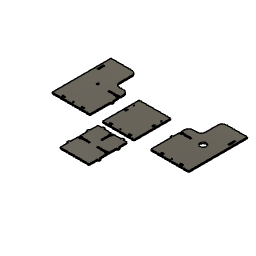
NEW housing (Autodesk Fusion 360 design; units mm, degrees)
Autodesk Fusion 360 part; units mm, degrees
note: some values were not read from the file. Set by a fixed rule: which sketch regions a step uses.
sketch "Sketch1" plane through (0, 0, 0) normal (0, 0, 1) x (1, 0, 0)
  line L0 (-200, 150) -> (-200, 236)
  line L1 (-196, 240) -> (-170, 240)
  line L2 (-160, 230) -> (-160, 225)
  line L3 (-150, 215) -> (-149.9799, 215)
  line L4 (-140, 150) -> (-200, 150)
  arc A0 (-160, 230) -> (-170, 240) centre (-170, 230) ccw
  arc A1 (-160, 225) -> (-150, 215) centre (-150, 225) ccw
  arc A2 (-140, 205) -> (-149.9799, 215) centre (-150, 205) ccw
  arc A3 (-196, 240) -> (-200, 236) centre (-196, 236) ccw
  circle A4 centre (-170, 192.9999) radius 2.5
  line L5 (-140, 205) -> (-140, 204.0941)
  line L6 (-140, 199.6441) -> (-140, 189.8941)
  line L7 (-140, 185.8941) -> (-140, 150)
  line L8 (-155, 153) -> (-155, 154.55)
  line L9 (-155, 154.55) -> (-149, 154.55)
  line L10 (-149, 154.55) -> (-149, 151.45)
  line L11 (-149, 151.45) -> (-155, 151.45)
  line L12 (-155, 151.45) -> (-155, 153)
  line L13 (-185, 153) -> (-185, 154.55)
  line L14 (-185, 154.55) -> (-191, 154.55)
  line L15 (-191, 154.55) -> (-191, 151.45)
  line L16 (-191, 151.45) -> (-185, 151.45)
  line L17 (-185, 151.45) -> (-185, 153)
  circle A5 centre (-170, 153) radius 1.5
  line L18 (-140, 202.9941) -> (-140, 204.0941)
  line L19 (-140, 189.8941) -> (-137.2, 189.8941)
  line L20 (-137.2, 189.8941) -> (-137.2, 185.8941)
  line L21 (-137.2, 185.8941) -> (-140, 185.8941)
  line L22 (-50, 150) -> (10, 150)
  line L23 (-35, 154.55) -> (-41, 154.55)
  line L24 (-52.8, 189.8941) -> (-52.8, 185.8941)
  line L25 (1, 151.45) -> (-5, 151.45)
  line L26 (1, 154.55) -> (1, 151.45)
  arc A6 (-40.0001, 215) -> (-50, 205) centre (-40, 205) ccw
  circle A7 centre (-20, 153) radius 1.5
  line L27 (-5, 154.55) -> (1, 154.55)
  line L28 (-52.8, 185.8941) -> (-50, 185.8941)
  line L29 (-50, 202.9941) -> (-50, 204.0941)
  line L30 (-39.9999, 215) -> (-40.0001, 215)
  line L31 (-41, 154.55) -> (-41, 151.45)
  arc A8 (10, 236) -> (6, 240) centre (6, 236) ccw
  line L32 (-50, 189.8941) -> (-52.8, 189.8941)
  line L33 (-41, 151.45) -> (-35, 151.45)
  line L34 (-50, 205) -> (-50, 204.0941)
  arc A9 (-39.9999, 215) -> (-30, 225) centre (-40, 225) ccw
  arc A10 (-20, 240) -> (-30, 230) centre (-20, 230) ccw
  line L35 (10, 150) -> (10, 236)
  line L36 (-50, 199.6441) -> (-50, 189.8941)
  line L37 (6, 240) -> (-20, 240)
  line L38 (-30, 230) -> (-30, 225)
  line L39 (-35, 153) -> (-35, 154.55)
  line L40 (-5, 153) -> (-5, 154.55)
  line L41 (-35, 151.45) -> (-35, 153)
  line L42 (-50, 185.8941) -> (-50, 150)
  line L43 (-5, 151.45) -> (-5, 153)
  line L44 (-77, 154.55) -> (-71, 154.55)
  line L45 (-77, 153) -> (-77, 154.55)
  line L46 (-77, 151.45) -> (-77, 153)
  line L47 (-71, 151.45) -> (-77, 151.45)
  line L48 (-71, 154.55) -> (-71, 151.45)
  circle A11 centre (-92, 153) radius 1.5
  line L49 (-107, 154.55) -> (-113, 154.55)
  line L50 (-107, 151.45) -> (-107, 153)
  line L51 (-107, 153) -> (-107, 154.55)
  line L52 (-113, 151.45) -> (-107, 151.45)
  line L53 (-113, 154.55) -> (-113, 151.45)
  circle A12 centre (-58.5, 201.1441) radius 1.55
  line L54 (-125, -50) -> (-55, -50)
  line L55 (-110.1464, 10) -> (-110.1464, 12.8)
  line L56 (-110.1464, 12.8) -> (-106, 12.8)
  line L57 (-106, 12.8) -> (-106, 10)
  line L58 (-73.9655, 10) -> (-73.9655, 12.8)
  line L59 (-73.9655, 12.8) -> (-69.9655, 12.8)
  line L60 (-69.9655, 12.8) -> (-69.9655, 10)
  line L61 (-91.55, 10) -> (-106, 10)
  line L62 (-110.1464, 10) -> (-125, 10)
  line L63 (-55, 10) -> (-69.9655, 10)
  line L64 (-73.9655, 10) -> (-88.45, 10)
  line L65 (-125, 0.1142) -> (-127.8, 0.1142)
  line L66 (-127.8, 0.1142) -> (-127.8, -3.8858)
  line L67 (-127.8, -3.8858) -> (-125, -3.8858)
  line L68 (-125, -35.6734) -> (-127.8, -35.6734)
  line L69 (-127.8, -35.6734) -> (-127.8, -39.6734)
  line L70 (-127.8, -39.6734) -> (-125, -39.6734)
  line L71 (-125, -39.6734) -> (-125, -50)
  line L72 (-125, 10) -> (-125, 0.1142)
  line L73 (-125, -3.8858) -> (-125, -18.27)
  line L74 (-125, -21.37) -> (-125, -35.6734)
  line L75 (-55, -21.37) -> (-55, -35.6734)
  line L76 (-55, -35.6734) -> (-52.2, -35.6734)
  line L77 (-52.2, -3.8858) -> (-55, -3.8858)
  line L78 (-52.2, -35.6734) -> (-52.2, -39.6734)
  line L79 (-55, 0.1142) -> (-52.2, 0.1142)
  line L80 (-52.2, 0.1142) -> (-52.2, -3.8858)
  line L81 (-55, -3.8858) -> (-55, -18.27)
  line L82 (-52.2, -39.6734) -> (-55, -39.6734)
  line L83 (-55, 0.1142) -> (-55, 10)
  line L84 (-55, -18.27) -> (-55, -3.8858)
  line L85 (-55, -50) -> (-55, -39.6734)
  line L86 (-55, -35.6734) -> (-55, -21.37)
  circle A13 centre (-20, 192.9999) radius 7.5
  circle A14 centre (-125.5, 201.1441) radius 1.55
  line L87 (-50, 202.9941) -> (-50, 202.6547)
  line L88 (-48, 202.6547) -> (-48, 204.5941)
  line L89 (-48, 204.5941) -> (-45.2, 204.5941)
  line L90 (-45.2, 204.5941) -> (-45.2, 202.6547)
  line L91 (-38.2, 202.3941) -> (-38.2, 199.8941)
  line L92 (-45.2, 199.6441) -> (-45.2, 197.6942)
  line L93 (-45.2, 197.6942) -> (-48, 197.6942)
  line L94 (-48, 197.6942) -> (-47.9999, 197.6942)
  line L95 (-47.9999, 197.6942) -> (-47.9999, 199.6441)
  line L96 (-141.9995, 202.6547) -> (-141.9995, 204.5941)
  line L97 (-141.9995, 204.5941) -> (-144.7995, 204.5941)
  line L98 (-151.7995, 202.3941) -> (-151.7995, 199.8941)
  line L99 (-144.7995, 199.8942) -> (-144.7995, 199.8941)
  line L100 (-144.7995, 197.6942) -> (-141.9995, 197.6942)
  line L101 (-141.9996, 197.6942) -> (-141.9996, 199.6441)
  line L102 (-140, 199.8941) -> (-139.9995, 199.8941)
  line L103 (-120.2005, -16.4059) -> (-120.2005, -16.4093)
  line L104 (-123.0005, -16.4059) -> (-120.2005, -16.4059)
  line L105 (-123.0005, -18.3593) -> (-123.0005, -16.4059)
  line L106 (-123.0004, -23.3058) -> (-123.0004, -21.3699)
  line L107 (-120.2005, -23.3058) -> (-123.0005, -23.3058)
  line L108 (-113.2005, -18.6059) -> (-113.2005, -21.1059)
  line L109 (-125, -21.37) -> (-125, -21.3699)
  line L110 (-56.9995, -18.3593) -> (-56.9995, -16.4059)
  line L111 (-56.9995, -16.4059) -> (-59.7995, -16.4059)
  line L112 (-59.7995, -16.4059) -> (-59.7995, -16.4093)
  line L113 (-66.7995, -18.6059) -> (-66.7995, -21.1059)
  line L114 (-59.7995, -23.3058) -> (-56.9995, -23.3058)
  line L115 (-56.9996, -23.3058) -> (-56.9996, -21.3699)
  line L116 (-55, -21.3699) -> (-55, -21.37)
  line L117 (-88.5262, 7.9998) -> (-86.5618, 7.9998)
  line L118 (-86.5618, 7.9998) -> (-86.5618, 5.1998)
  line L119 (-86.5618, 5.1998) -> (-86.5902, 5.1998)
  line L120 (-88.7618, -1.8002) -> (-91.2618, -1.8002)
  line L121 (-93.4618, 5.1998) -> (-93.4618, 7.9998)
  line L122 (-93.4618, 7.9997) -> (-91.5368, 7.9997)
  line L123 (-91.2618, 9.9998) -> (-91.55, 10)
  line L124 (-50, 202.6547) -> (-48, 202.6547)
  line L125 (-45.2, 202.6547) -> (-38.2, 202.6547)
  line L126 (-38.2, 202.6547) -> (-38.2, 202.3941)
  line L127 (-50, 199.6441) -> (-47.9999, 199.6441)
  line L128 (-45.2, 199.6441) -> (-38.2, 199.6441)
  line L129 (-38.2, 199.6441) -> (-38.2, 199.8941)
  line L130 (-144.8, 202.6547) -> (-151.8, 202.6547)
  line L131 (-144.8, 199.6441) -> (-151.8, 199.6441)
  line L132 (-144.8, 199.6441) -> (-144.8, 197.6942)
  line L133 (-144.8, 197.6942) -> (-142, 197.6942)
  line L134 (-142.0001, 197.6942) -> (-142.0001, 199.6441)
  line L135 (-140, 199.6441) -> (-142.0001, 199.6441)
  line L136 (-140, 202.6547) -> (-142, 202.6547)
  line L137 (-142, 202.6547) -> (-142, 204.5941)
  line L138 (-142, 204.5941) -> (-144.8, 204.5941)
  line L139 (-144.8, 204.5941) -> (-144.8, 202.6547)
  line L140 (-151.8, 202.6547) -> (-151.8, 202.3941)
  line L141 (-151.8, 199.6441) -> (-151.8, 199.8941)
  line L142 (-56.9995, -23.3093) -> (-59.7995, -23.3093)
  line L143 (-56.9995, -21.3699) -> (-56.9995, -23.3093)
  line L144 (-55, -21.3699) -> (-57, -21.3699)
  line L145 (-55, -18.3593) -> (-57.0001, -18.3593)
  line L146 (-57.0001, -16.4093) -> (-57.0001, -18.3593)
  line L147 (-59.7995, -16.4093) -> (-56.9995, -16.4093)
  line L148 (-59.8, -18.3593) -> (-59.8, -16.4093)
  line L149 (-59.8, -18.3593) -> (-66.8, -18.3593)
  line L150 (-66.7995, -21.1093) -> (-66.7995, -18.6093)
  line L151 (-59.8, -21.3699) -> (-66.8, -21.3699)
  line L152 (-66.8, -21.3699) -> (-66.8, -21.1093)
  line L153 (-66.8, -18.3593) -> (-66.8, -18.6093)
  line L154 (-140, 202.9941) -> (-140, 202.6547)
  line L155 (-59.7995, -23.3058) -> (-59.8, -21.3699)
  line L156 (-55, -18.27) -> (-55, -18.3593)
  line L157 (-120.2, -18.3593) -> (-113.2, -18.3593)
  line L158 (-120.2, -18.3593) -> (-120.2, -16.4093)
  line L159 (-120.2005, -16.4093) -> (-123.0005, -16.4093)
  line L160 (-122.9999, -16.4093) -> (-122.9999, -18.3593)
  line L161 (-125, -18.3593) -> (-122.9999, -18.3593)
  line L162 (-125, -21.3699) -> (-123, -21.3699)
  line L163 (-123.0005, -21.3699) -> (-123.0005, -23.3093)
  line L164 (-123.0005, -23.3093) -> (-120.2005, -23.3093)
  line L165 (-120.2005, -23.3058) -> (-120.2, -21.3699)
  line L166 (-120.2, -21.3699) -> (-113.2, -21.3699)
  line L167 (-113.2005, -21.1093) -> (-113.2005, -18.6093)
  line L168 (-113.2, -18.3593) -> (-113.2, -18.6093)
  line L169 (-113.2, -21.3699) -> (-113.2, -21.1093)
  line L170 (-91.5368, 9.9991) -> (-91.5368, 7.999)
  line L171 (-93.4868, 7.999) -> (-91.5368, 7.999)
  line L172 (-93.4868, 5.1996) -> (-93.4868, 7.9996)
  line L173 (-91.5368, 5.1991) -> (-93.4868, 5.1992)
  line L174 (-91.5368, 5.1991) -> (-91.5368, -1.8009)
  line L175 (-88.7868, -1.8004) -> (-91.2868, -1.8004)
  line L176 (-88.5262, 5.1991) -> (-88.5262, -1.8009)
  line L177 (-86.5902, 5.1996) -> (-88.5262, 5.1991)
  line L178 (-86.5902, 5.1996) -> (-86.5902, 7.9996)
  line L179 (-88.5262, 7.9996) -> (-86.5868, 7.9996)
  line L180 (-88.5262, 9.9991) -> (-88.5262, 7.9991)
  line L181 (-91.5368, -1.8009) -> (-91.2868, -1.8009)
  line L182 (-88.5262, -1.8009) -> (-88.7868, -1.8009)
  line L183 (-130, 150) -> (-54, 150)
  line L184 (-54, 150) -> (-54, 220)
  line L185 (-54, 220) -> (-130, 220)
  line L186 (-130, 220) -> (-130, 150)
  point P0 (-200, 240)
  point P1 (-160, 240)
  point P2 (-160, 215)
  point P3 (-140, 214.9799)
  point P4 (-50, 214.9999)
  point P5 (10, 240)
  point P6 (-30, 215)
  point P7 (-30, 240)
  point P8 (-122, 101.4441)
  dimension "d1" = 90
  dimension "d2" = 40
  dimension "d3" = 25
  dimension "d4" = 20
  dimension "d5" = 10
  dimension "d6" = 4
  dimension "d7" = 5
  dimension "d17" = 15
  dimension "d18" = 1.55
  dimension "d19" = 6
  dimension "d20" = 3.1
  dimension "d21" = 3
  dimension "d30" = 2.8
  dimension "d31" = 4
  dimension "d34" = 3.1
  dimension "d41" = 2.8
  dimension "d42" = 4
  dimension "d52" = 2.8
  dimension "d53" = 4
  dimension "d54" = 2.8
  dimension "d55" = 4
  dimension "d56" = 15
  dimension "d67" = 2.8
  dimension "d74" = 76
  dimension "d75" = 70
  constraint vertical L0
  constraint perpendicular L0 L1
  constraint perpendicular L1 L2
  constraint perpendicular L1 L5
  constraint perpendicular L0 L4
  constraint coincident P1 L1
  constraint coincident P1 L2
  constraint tangent L1 A0
  constraint tangent L2 A0
  constraint coincident P2 L2
  constraint tangent L2 A1
  constraint equal A0 A1
  constraint coincident P3 L3
  constraint coincident P3 L5
  constraint tangent L3 A2
  constraint tangent A2 L5
  constraint equal A0 A2
  constraint coincident P0 L0
  constraint coincident P0 L1
  constraint tangent L0 A3
  constraint tangent L1 A3
  constraint coincident L102.start L5
  constraint collinear L5 L6
  constraint coincident L7.start L6
  constraint collinear L6 L7
  constraint perpendicular L4 L10
  constraint perpendicular L19 L20
  constraint perpendicular L63 L72
  constraint perpendicular L54 L72
  constraint perpendicular L54 L85
  constraint coincident L55.start L63
  constraint perpendicular L55 L63
  constraint coincident L57.end L63
  constraint perpendicular L57 L63
  constraint coincident L58.start L63
  constraint perpendicular L58 L63
  constraint perpendicular L58 L59
  constraint perpendicular L60 L63
  constraint coincident L61.start L63
  constraint collinear L61 L63
  constraint collinear L61 L62
  constraint collinear L63 L64
  constraint perpendicular L65 L72
  constraint perpendicular L65 L66
  constraint coincident L67.end L72
  constraint perpendicular L67 L72
  constraint perpendicular L68 L72
  constraint perpendicular L68 L69
  constraint coincident L70.end L72
  constraint perpendicular L70 L72
  constraint collinear L71 L72
  constraint collinear L72 L73
  constraint collinear L73 L74
  constraint collinear L83 L85
  constraint collinear L84 L85
  constraint collinear L85 L86
  constraint perpendicular L88 L93
  constraint perpendicular L93 L95
  constraint perpendicular L88 L124
  constraint perpendicular L91 L125
  constraint perpendicular L95 L127
  constraint perpendicular L91 L128
  constraint parallel L91 L129
  constraint coincident L136 L96.start
  constraint coincident L135 L101.end
  constraint coincident L145 L110.start
  constraint coincident L144 L115.end
  constraint coincident L161 L105.start
  constraint coincident L162 L106.end
  constraint coincident L178 L119.end
  constraint coincident L180 L117.start
  constraint coincident L170 L122.end
  constraint horizontal L183
  constraint perpendicular L184 L185
  constraint perpendicular L183 L186
  measures "d1" distance of L0.start P0
  measures "d2" distance of P0 P1
  measures "d3" distance of P1 P2
  measures "d4" distance of P2 P3
  measures "d5" radius of A0
  measures "d6" radius of A3
  measures "d7" diameter of A4
  measures "d17" distance of L8.start A5.centre
  measures "d18" distance of L8.start L8.end
  measures "d19" distance of L8.end L9.end
  measures "d20" distance of L9.end L10.end
  measures "d21" diameter of A5
  measures "d30" distance of L6.end L19.end
  measures "d31" distance of L19.end L20.end
  measures "d34" diameter of A12
  measures "d41" distance of L55.start L55.end
  measures "d42" distance of L58.end L59.end
  measures "d52" distance of L65.start L65.end
  measures "d53" distance of L65.end L66.end
  measures "d54" distance of L68.start L68.end
  measures "d55" distance of L68.end L69.end
  measures "d56" diameter of A13
  measures "d67" distance of L88.end L89.end
  measures "d74" distance of L183.start L183.end
  measures "d75" distance of L183.end L184.end
sketch "Sketch2" plane through (0, 0, 0) normal (0, 0, 1) x (1, 0, 0)
  line L0 (-125, 125) -> (-127, 125)
  line L1 (-127, 125) -> (-127, 128)
  line L2 (-127, 128) -> (-125, 128)
  line L3 (-125, 128) -> (-125, 129.5)
  line L4 (-125, 129.5) -> (-55, 129.5)
  line L5 (-55, 129.5) -> (-55, 128)
  line L6 (-55, 128) -> (-52, 128)
  line L7 (-52, 128) -> (-52, 125)
  line L8 (-52, 125) -> (-55, 125)
  line L9 (-55, 125) -> (-55, 123.5)
  line L10 (-55, 123.5) -> (-125, 123.5)
  line L11 (-125, 123.5) -> (-125, 125)
  line L12 (-197, 225) -> (-197, 220)
  line L13 (-197, 220) -> (-194, 220)
  line L14 (-194, 220) -> (-194, 225)
  line L15 (-194, 225) -> (-197, 225)
  line L16 (4, 225) -> (7, 225)
  line L17 (7, 225) -> (7, 220)
  line L18 (7, 220) -> (4, 220)
  line L19 (4, 220) -> (4, 225)
  dimension "d59" = 3
  dimension "d60" = 1.5
  dimension "d61" = 3
  constraint horizontal L0
  constraint perpendicular L0 L1
  constraint perpendicular L1 L2
  constraint perpendicular L2 L3
  constraint perpendicular L1 L4
  constraint perpendicular L4 L5
  constraint perpendicular L5 L6
  constraint perpendicular L0 L7
  constraint perpendicular L7 L8
  constraint perpendicular L8 L9
  constraint perpendicular L9 L10
  constraint perpendicular L0 L11
  constraint vertical L12
  constraint perpendicular L12 L13
  constraint perpendicular L13 L14
  constraint perpendicular L12 L15
  measures "d59" distance of L5.end L6.end
  measures "d60" distance of L8.end L9.end
  measures "d61" distance of L12.end L13.end
sketch "Sketch4" plane through (0, 0, 0) normal (0, 0, 1) x (1, 0, 0)
  line L0 (-115.3, 202.6) -> (-115.3, 199.7)
  constraint vertical L0
sketch "Sketch5" plane through (0, 0, 0) normal (0, 0, 1) x (1, 0, 0)
  line L0 (5, 410) -> (55, 410)
  line L1 (55, 410) -> (55, 275)
  line L2 (-5, 400) -> (-5, 370)
  line L3 (-15, 360) -> (-25, 360)
  arc A0 (5, 410) -> (-5, 400) centre (5, 400) ccw
  arc A1 (-15, 360) -> (-5, 370) centre (-15, 370) ccw
  arc A2 (-25, 360) -> (-35, 350) centre (-25, 350) ccw
  line L4 (-35, 341.3537) -> (-32, 341.3537)
  line L5 (-32, 341.3537) -> (-32, 343.0537)
  line L6 (-32, 343.0537) -> (-29.4, 343.0537)
  line L7 (-29.4, 343.0537) -> (-29.4, 341.3537)
  line L8 (-29.4, 341.3537) -> (-9.4, 341.3537)
  line L9 (-9.4, 341.3537) -> (-9.4, 338.3537)
  line L10 (-9.4, 338.3537) -> (-29.4, 338.3537)
  line L11 (-29.4, 338.3537) -> (-29.4, 336.6537)
  line L12 (-29.4, 336.6537) -> (-32, 336.6537)
  line L13 (-32, 336.6537) -> (-32, 338.3537)
  line L14 (-32, 338.3537) -> (-35, 338.3537)
  line L15 (-35, 341.3537) -> (-35, 350)
  line L16 (-35, 324.1422) -> (-38, 324.1422)
  line L17 (-38, 324.1422) -> (-38, 319.1422)
  line L18 (-38, 319.1422) -> (-35, 319.1422)
  line L19 (-35, 275) -> (-35, 319.1422)
  line L20 (-35, 324.1422) -> (-35, 338.3537)
  circle A3 centre (18, 341.6537) radius 7.475
  circle A4 centre (10, 275) radius 1.5
  line L21 (30, 275) -> (30, 276.55)
  line L22 (30, 276.55) -> (36, 276.55)
  line L23 (36, 276.55) -> (36, 273.55)
  line L24 (36, 273.55) -> (30, 273.55)
  line L25 (30, 273.55) -> (30, 275)
  line L26 (-10, 275) -> (-10, 276.55)
  line L27 (-16, 276.55) -> (-16, 273.55)
  line L28 (-16, 273.55) -> (-10, 273.55)
  line L29 (-10, 273.55) -> (-10, 275)
  line L30 (-270, 410) -> (-270, 270)
  line L31 (-180, 324.1422) -> (-180, 338.3537)
  arc A5 (-210, 370) -> (-200, 360) centre (-200, 370) ccw
  line L32 (-199, 276.55) -> (-199, 273.55)
  line L33 (-205, 273.55) -> (-205, 275)
  line L34 (-251, 276.55) -> (-251, 273.55)
  line L35 (-220, 410) -> (-270, 410)
  line L36 (-245, 273.55) -> (-245, 275)
  line L37 (-180, 270) -> (-180, 319.1422)
  line L38 (-185.6, 338.3537) -> (-185.6, 336.6537)
  line L39 (-199, 273.55) -> (-205, 273.55)
  line L40 (-185.6, 336.6537) -> (-183, 336.6537)
  line L41 (-210, 400) -> (-210, 370)
  line L42 (-205.6, 338.3537) -> (-185.6, 338.3537)
  line L43 (-245, 276.55) -> (-251, 276.55)
  line L44 (-177, 319.1422) -> (-180, 319.1422)
  line L45 (-270, 270) -> (-180, 270)
  circle A6 centre (-225, 275) radius 1.5
  line L46 (-180, 341.3537) -> (-183, 341.3537)
  line L47 (-205, 275) -> (-205, 276.55)
  line L48 (-205, 276.55) -> (-199, 276.55)
  line L49 (-245, 275) -> (-245, 276.55)
  arc A7 (-210, 400) -> (-220, 410) centre (-220, 400) ccw
  line L50 (-251, 273.55) -> (-245, 273.55)
  line L51 (-177, 324.1422) -> (-177, 319.1422)
  line L52 (-183, 336.6537) -> (-183, 338.3537)
  line L53 (-183, 343.0537) -> (-185.6, 343.0537)
  line L54 (-205.6, 341.3537) -> (-205.6, 338.3537)
  line L55 (-185.6, 341.3537) -> (-205.6, 341.3537)
  line L56 (-180, 324.1422) -> (-177, 324.1422)
  line L57 (-183, 338.3537) -> (-180, 338.3537)
  arc A8 (-180, 350) -> (-190, 360) centre (-190, 350) ccw
  line L58 (-200, 360) -> (-190, 360)
  line L59 (-180, 341.3537) -> (-180, 350)
  line L60 (-183, 341.3537) -> (-183, 343.0537)
  line L61 (-185.6, 343.0537) -> (-185.6, 341.3537)
  circle A9 centre (-233, 341.6537) radius 2.475
  line L62 (-150, 270) -> (-75, 270)
  line L63 (-75, 270) -> (-75, 357.0711)
  line L64 (-75, 357.0711) -> (-75.0001, 357.0711)
  line L65 (-75.0001, 357.0711) -> (-150.0001, 357.0711)
  line L66 (-150.0001, 357.0711) -> (-150, 270)
  circle A10 centre (-145.0001, 339.8537) radius 1.5
  line L67 (-146.5501, 324.3142) -> (-145.0001, 324.3142)
  line L68 (-145.0001, 324.3142) -> (-143.4501, 324.3142)
  line L69 (-143.4501, 324.3142) -> (-145.0001, 324.3142)
  line L70 (-143.4501, 324.3142) -> (-143.4501, 318.9182)
  line L71 (-143.4501, 318.9182) -> (-146.5501, 318.9182)
  line L72 (-146.5501, 318.9182) -> (-146.5501, 324.3142)
  line L73 (-81.5501, 318.9182) -> (-78.4501, 318.9182)
  line L74 (-78.4501, 324.3142) -> (-80.0001, 324.3142)
  line L75 (-80.0001, 324.3142) -> (-81.5501, 324.3142)
  circle A11 centre (-80.0001, 339.8537) radius 1.5
  line L76 (-81.5501, 324.3142) -> (-80.0001, 324.3142)
  line L77 (-78.4501, 318.9182) -> (-78.4501, 324.3142)
  line L78 (-81.5501, 324.3142) -> (-81.5501, 318.9182)
  line L79 (-132.4853, 276.55) -> (-138.4853, 276.55)
  line L80 (-92.4853, 275) -> (-92.4853, 276.55)
  line L81 (-86.4853, 273.55) -> (-92.4853, 273.55)
  line L82 (-132.4853, 275) -> (-132.4853, 276.55)
  line L83 (-92.4853, 276.55) -> (-86.4853, 276.55)
  line L84 (-138.4853, 273.55) -> (-132.4853, 273.55)
  line L85 (-132.4853, 273.55) -> (-132.4853, 275)
  line L86 (-86.4853, 276.55) -> (-86.4853, 273.55)
  line L87 (-92.4853, 273.55) -> (-92.4853, 275)
  circle A12 centre (-112.4853, 275) radius 1.5
  line L88 (-138.4853, 276.55) -> (-138.4853, 273.55)
  line L89 (-78.0463, 165.9537) -> (-147.0463, 165.9537)
  line L90 (-144.1, 212.4537) -> (-144.1, 214.1537)
  line L91 (-141.5, 207.7537) -> (-144.1, 207.7537)
  line L92 (-121.5, 212.4537) -> (-121.5, 209.4537)
  line L93 (-144.1, 207.7537) -> (-144.1, 209.4537)
  line L94 (-144.1, 209.4537) -> (-147.1, 209.4537)
  line L95 (-144.1, 214.1537) -> (-141.5, 214.1537)
  line L96 (-141.5, 209.4537) -> (-141.5, 207.7537)
  line L97 (-141.5, 214.1537) -> (-141.5, 212.4537)
  line L98 (-147.1, 212.4537) -> (-144.1, 212.4537)
  line L99 (-121.5, 209.4537) -> (-141.5, 209.4537)
  line L100 (-141.5, 212.4537) -> (-121.5, 212.4537)
  line L101 (-147.0463, 231.2674) -> (-150.0463, 231.2674)
  line L102 (-150.0463, 231.2674) -> (-150.0463, 236.7974)
  line L103 (-150.0463, 236.7974) -> (-147.0463, 236.7974)
  line L104 (-147.0463, 212.4537) -> (-147.0463, 231.2674)
  line L105 (-147.0463, 236.7974) -> (-147.0463, 255.9537)
  line L106 (-150.0464, 185.2375) -> (-147.0464, 185.2375)
  line L107 (-147.0464, 190.7674) -> (-150.0464, 190.7674)
  line L108 (-150.0464, 190.7674) -> (-150.0464, 185.2375)
  line L109 (-147.0463, 165.9537) -> (-147.0464, 185.2375)
  line L110 (-147.0464, 190.7674) -> (-147.0463, 209.4537)
  line L111 (-92.0699, 255.9537) -> (-92.0699, 258.9537)
  line L112 (-92.0699, 258.9537) -> (-86.7161, 258.9537)
  line L113 (-86.7161, 258.9537) -> (-86.7161, 255.9537)
  line L114 (-138.2447, 255.9537) -> (-138.2447, 258.9537)
  line L115 (-138.2447, 258.9537) -> (-132.7, 258.9537)
  line L116 (-132.7, 258.9537) -> (-132.7, 255.9537)
  line L117 (-147.0463, 255.9537) -> (-138.2447, 255.9537)
  line L118 (-86.7161, 255.9537) -> (-78.0463, 255.9537)
  line L119 (-115.75, 252.9537) -> (-115.75, 250.3537)
  line L120 (-111.05, 230.3537) -> (-111.05, 250.3537)
  line L121 (-115.75, 250.3537) -> (-114.05, 250.3537)
  line L122 (-111.05, 250.3537) -> (-109.35, 250.3537)
  line L123 (-111.05, 252.9537) -> (-111.05, 255.9537)
  line L124 (-114.05, 255.9537) -> (-114.05, 252.9537)
  line L125 (-109.35, 250.3537) -> (-109.35, 252.9537)
  line L126 (-114.05, 230.3537) -> (-111.05, 230.3537)
  line L127 (-109.35, 252.9537) -> (-111.05, 252.9537)
  line L128 (-114.05, 252.9537) -> (-115.75, 252.9537)
  line L129 (-114.05, 250.3537) -> (-114.05, 230.3537)
  line L130 (-132.7, 255.9537) -> (-114.05, 255.9537)
  line L131 (-111.05, 255.9537) -> (-92.0699, 255.9537)
  line L132 (-75.0463, 231.2674) -> (-75.0463, 236.7974)
  line L133 (-83.5927, 207.7537) -> (-80.9927, 207.7537)
  line L134 (-80.9927, 207.7537) -> (-80.9927, 209.4537)
  line L135 (-83.5927, 214.1537) -> (-83.5927, 212.4537)
  line L136 (-78.0463, 212.4537) -> (-78.0463, 231.2674)
  line L137 (-77.9927, 212.4537) -> (-80.9927, 212.4537)
  line L138 (-103.5927, 212.4537) -> (-103.5927, 209.4537)
  line L139 (-80.9927, 209.4537) -> (-77.9927, 209.4537)
  line L140 (-80.9927, 212.4537) -> (-80.9927, 214.1537)
  line L141 (-75.0463, 236.7974) -> (-78.0463, 236.7974)
  line L142 (-78.0463, 231.2674) -> (-75.0463, 231.2674)
  line L143 (-83.5927, 209.4537) -> (-83.5927, 207.7537)
  line L144 (-78.0463, 190.7674) -> (-75.0463, 190.7674)
  line L145 (-80.9927, 214.1537) -> (-83.5927, 214.1537)
  line L146 (-75.0463, 185.2375) -> (-78.0463, 185.2375)
  line L147 (-75.0463, 190.7674) -> (-75.0463, 185.2375)
  line L148 (-78.0463, 190.7674) -> (-78.0463, 209.4537)
  line L149 (-103.5927, 209.4537) -> (-83.5927, 209.4537)
  line L150 (-83.5927, 212.4537) -> (-103.5927, 212.4537)
  line L151 (-78.0463, 255.9537) -> (-78.0463, 236.7974)
  line L152 (-78.0463, 231.2674) -> (-78.0463, 212.4537)
  line L153 (-78.0463, 209.4537) -> (-78.0463, 190.7674)
  line L154 (-78.0463, 185.2375) -> (-78.0463, 165.9537)
  line L155 (-265, 387) -> (-262, 387)
  line L156 (-262, 387) -> (-262, 372)
  line L157 (-262, 372) -> (-265, 372)
  line L158 (-265, 372) -> (-265, 387)
  line L159 (50, 372) -> (50, 387)
  line L160 (47, 387) -> (47, 372)
  line L161 (47, 372) -> (50, 372)
  line L162 (50, 387) -> (47, 387)
  line L163 (10, 275) -> (10, 273.5)
  line L164 (10, 270) -> (55, 270)
  line L165 (55, 270) -> (55, 275)
  line L166 (-35, 275) -> (-35, 270)
  line L167 (-35, 270) -> (10, 270)
  line L168 (11.5, 275) -> (8.5, 275)
  line L169 (-16, 276.55) -> (-10, 276.55)
  point P0 (-114.05, 255.9)
  point P1 (-111.05, 255.9)
  dimension "d84" = 10
  dimension "d90" = 3
  dimension "d91" = 1.7
  dimension "d92" = 2.6
  dimension "d93" = 20
  dimension "d94" = 3
  dimension "d95" = 1.7
  dimension "d96" = 3
  dimension "d97" = 5
  dimension "d98" = 14.95
  dimension "d100" = 3
  dimension "d102" = 1.55
  dimension "d103" = 6
  dimension "d104" = 3
  dimension "d106" = 4.95
  dimension "d107" = 75
  dimension "d109" = 3
  dimension "d111" = 1.55
  dimension "d112" = 3.1
  dimension "d114" = 69
  dimension "d115" = 3
  dimension "d117" = 3
  dimension "d118" = 3
  dimension "d124" = 3
  dimension "d125" = 15
  dimension "d126" = 5
  dimension "d127" = 5
  constraint vertical L19
  constraint perpendicular L0 L19
  constraint perpendicular L0 L1
  constraint perpendicular L0 L2
  constraint perpendicular L3 L19
  constraint tangent L2 A0
  constraint tangent L0 A0
  constraint tangent L2 A1
  constraint tangent L3 A1
  constraint equal A0 A1
  constraint tangent L3 A2
  constraint tangent A2 L19
  constraint equal A0 A2
  constraint coincident L4.start L19
  constraint perpendicular L4 L19
  constraint perpendicular L5 L8
  constraint perpendicular L8 L9
  constraint perpendicular L7 L10
  constraint perpendicular L10 L11
  constraint perpendicular L5 L12
  constraint perpendicular L4 L13
  constraint perpendicular L14 L19
  constraint collinear L15 L19
  constraint coincident L16.start L19
  constraint perpendicular L16 L19
  constraint perpendicular L14 L17
  constraint perpendicular L18 L19
  constraint collinear L19 L20
  constraint perpendicular L21 L22
  constraint perpendicular L21 L24
  constraint horizontal L62
  constraint perpendicular L46 L63
  constraint perpendicular L63 L65
  constraint perpendicular L66 L67
  constraint perpendicular L66 L68
  constraint perpendicular L66 L69
  constraint perpendicular L70 L71
  constraint perpendicular L67 L72
  constraint perpendicular L109 L117
  constraint perpendicular L117 L151
  constraint perpendicular L89 L109
  constraint coincident L94 L110.end
  constraint coincident L98 L104.start
  constraint collinear L104 L109
  constraint perpendicular L101 L104
  constraint coincident L103.end L104
  constraint perpendicular L103 L104
  constraint collinear L104 L105
  constraint collinear L109 L110
  constraint coincident L111.start L117
  constraint perpendicular L111 L117
  constraint perpendicular L86 L112
  constraint coincident L113.end L117
  constraint perpendicular L113 L117
  constraint perpendicular L114 L117
  constraint perpendicular L85 L115
  constraint coincident L116.end L117
  constraint perpendicular L116 L117
  constraint collinear L117 L130
  constraint collinear L118 L130
  constraint collinear L130 L131
  constraint collinear L151 L153
  constraint collinear L151 L152
  constraint collinear L153 L154
  constraint horizontal L155
  constraint vertical L156
  constraint horizontal L157
  constraint vertical L158
  constraint coincident A4.centre L163.start
  constraint perpendicular L1 L164
  constraint vertical L165
  constraint coincident A4 L163.end
  constraint coincident A4 L168.end
  constraint coincident A4 L168.start
  constraint perpendicular L26 L169
  measures "d84" radius of A0
  measures "d90" distance of L4.start L4.end
  measures "d91" distance of L4.end L5.end
  measures "d92" distance of L5.end L6.end
  measures "d93" distance of L7.end L8.end
  measures "d94" distance of L8.end L9.end
  measures "d95" distance of L10.end L11.end
  measures "d96" distance of L16.start L16.end
  measures "d97" distance of L16.end L17.end
  measures "d98" diameter of A3
  measures "d100" diameter of A4
  measures "d102" distance of L21.start L21.end
  measures "d103" distance of L21.end L22.end
  measures "d104" distance of L22.end L23.end
  measures "d106" diameter of A9
  measures "d107" distance of L62.start L62.end
  measures "d109" diameter of A10
  measures "d111" distance of L67.end L68.end
  measures "d112" distance of L70.end L71.end
  measures "d114" distance of L105.end L118.end
  measures "d115" distance of L101.start L101.end
  measures "d117" distance of L111.start L111.end
  measures "d118" distance of L114.start L114.end
  measures "d124" distance of L155.start L155.end
  measures "d125" distance of L155.start L157.end
  measures "d126" distance of A4.centre L164.start
  measures "d127" distance of L19.start L166.end
extrude "Extrude1" add sketch "Sketch5" along normal blind 3 makes body 1 at (-112.5325, 304.7774, 0) makes body 2 at (43.381, 328.8168, 0) makes body 3 at (-256.7883, 327.6414, 0) makes body 4 at (-109.5618, 180.4537, 0)
sketch "Sketch3" plane through (0, 0, 0) normal (0, 0, 1) x (1, 0, 0)
equation "d112 = 1.55 mm + 1.55 mm"
